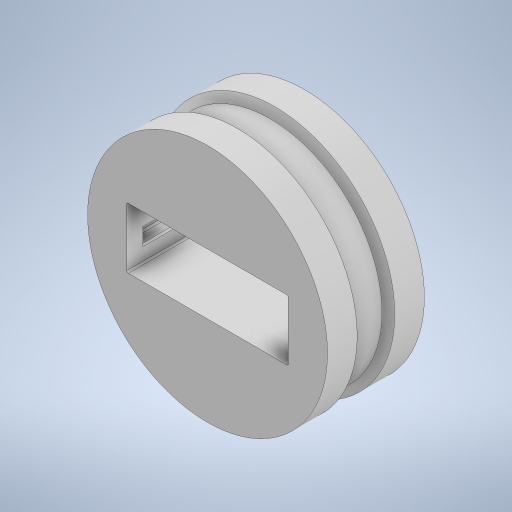
# Autodesk Inventor part: FMR_DXWD80_CPW_Halter_C_TdOS_Waveguide
Saved by Autodesk Inventor 2024.2 (Build 282272000, 272)
## iProperties
Created: 2023-05-10
Part Number: FMR_DXWD80_CPW_Halter_C_TdOS_Waveguide
Material: Generisch
Document SubType Name: Modeling
Designer: Markus Meinert
Density: 1 g/cm^3
Appearance: Vorgabe
Author: Markus Meinert
Autodesk Inventor part; units mm, degrees
ref_plane "YZ Plane" through (0, 0, 0) normal (1, 0, 0) x (0, 1, 0)
ref_plane "XZ Plane" through (0, 0, 0) normal (0, 1, 0) x (-1, 0, 0)
ref_plane "XY Plane" through (0, 0, 0) normal (0, 0, 1) x (1, 0, 0)
sketch "Skizze2" plane through (0, 0, 0) normal (0, 1, 0) x (-1, 0, 0)
  line L0 (0, -6) -> (-14.85, -6)
  line L1 (-14.85, -6) -> (-14.85, -2.3274)
  line L2 (-14.85, -2.3274) -> (-13.85, -1.75)
  line L3 (-13.85, -1.75) -> (-13.85, 1.75)
  line L4 (-13.85, 1.75) -> (-14.85, 2.3274)
  line L5 (-14.85, 2.3274) -> (-14.85, 6)
  line L6 (-14.85, 6) -> (0, 6)
  line L7 (0, 6) -> (0, -6)
  point P0 (0, 0)
  point P1 (-13.85, 0)
  point P2 (0, 0)
  dimension "d3" = 29.7
  dimension "d4" = 12
  dimension "d5" = 3.5
  dimension "d6" = 120
  dimension "d7" = 120
  dimension "d8" = 1
  constraints: 16 end point, 3 midpoint, 3 perpendicular, 2 point on line, 1 coincident, 1 horizontal, 1 horizontal alignment
  measures "d3" diameter of L1 L7
  measures "d4" distance between parallel lines of L6 L0
  measures "d5" distance of L2.end L3.end
  measures "d6" angle of L1 L2
  measures "d7" angle of L5 L4
  measures "d8" distance between parallel lines of L5 L3
revolve "Umdrehung1" add sketch "Skizze2" angle 360 about axis through (0, 0, 6) along (0, 0, -1)
sketch "Skizze3" plane through (0, 0, 6) normal (0, 0, 1) x (1, 0, 0)
  line L0 (-10, -3.75) -> (10, -3.75)
  line L1 (10, -3.75) -> (10, 3.75)
  line L2 (10, 3.75) -> (-10, 3.75)
  line L3 (-10, 3.75) -> (-10, -3.75)
  line L4 (-10, -3.75) -> (10, 3.75) construction
  line L5 (10, -3.75) -> (-10, 3.75) construction
  point P0 (0, 0)
  point P1 (0, 0)
  dimension "d10" = 20
  dimension "d11" = 7.5
  dimension "d12" = 0
  constraints: 12 end point, 2 midpoint, 2 parallel, 1 horizontal, 1 perpendicular
  measures "d10" distance of L2.end L1.end
  measures "d11" distance of L1.end L0.end
  measures "d12" distance of point (0, 0) point (0, 0)
extrude "Extrusion2" cut sketch "Skizze3" against normal through all
sketch "Skizze4" plane through (0, 0, -6) normal (0, 0, -1) x (-1, 0, 0)
  line L0 (-11.5, -1.8) -> (11.5, -1.8)
  line L1 (11.5, -1.8) -> (11.5, 0)
  line L2 (11.5, 0) -> (-11.5, 0)
  line L3 (-11.5, 0) -> (-11.5, -1.8)
  line L4 (-11.5, -1.8) -> (11.5, 0) construction
  line L5 (11.5, -1.8) -> (-11.5, 0) construction
  circle A0 centre (0, 0) radius 14.85 projected
  point P0 (0, -0.9)
  dimension "d15" = 23
  dimension "d16" = 1.8
  constraints: 12 end point, 3 midpoint, 2 parallel, 1 coincident, 1 horizontal, 1 perpendicular
  measures "d15" distance of L2.end L1.end
  measures "d16" distance of L1.end L0.end
extrude "Extrusion3" cut sketch "Skizze4" against normal blind 10 contours L3 L2 L1 L0
fillet "Rundung1" radius 0.2 4 edges at (10, -3.75, 0) (-10, -3.75, 0) (-10, 3.75, 0) (10, 3.75, 0)
fillet "Rundung2" radius 0.2 8 edges at (-10, -1.8, -1) (-11.5, -1.8, -1) (-11.5, 0, -1) (-10, 0, -1) (10, -1.8, -1) (11.5, -1.8, -1) (11.5, 0, -1) (10, 0, -1)
